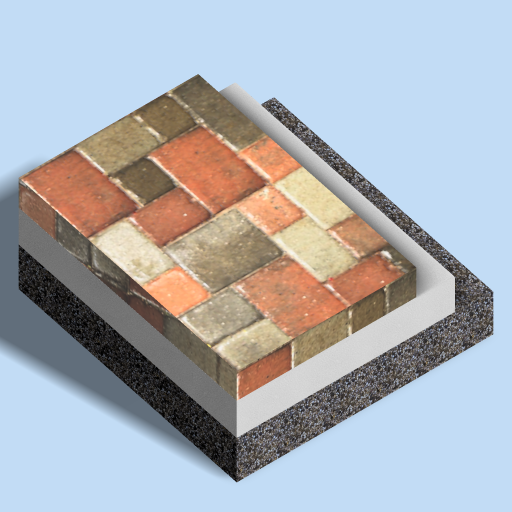
# Autodesk Inventor part: 부품1
Saved by Autodesk Inventor 2024.1 (Build 281209000, 209)
## iProperties
Created: 2024-01-18
Part Number: 부품1
Material: 일반
Document SubType Name: Modeling
Designer: likek
Density: 1 g/cm^3
Appearance: 기본값
Author: likek
Autodesk Inventor part; units mm, degrees
ref_plane "YZ Plane" through (0, 0, 0) normal (1, 0, 0) x (0, 1, 0)
ref_plane "XZ Plane" through (0, 0, 0) normal (0, 1, 0) x (-1, 0, 0)
ref_plane "XY Plane" through (0, 0, 0) normal (0, 0, 1) x (1, 0, 0)
sketch "스케치1" plane through (0, 0, 0) normal (0, 0, 1) x (1, 0, 0)
  line L0 (0, 0) -> (0, 150)
  line L1 (0, 150) -> (-850, 377.7568)
  line L2 (-850, 377.7568) -> (-850, 227.7568)
  line L3 (-850, 227.7568) -> (0, 0)
  line L4 (-311.1275, 0) -> (112.1526, 0)
  line L5 (-850, 377.7568) -> (-850, 602.7568)
  line L6 (-850, 602.7568) -> (0, 375)
  line L7 (0, 375) -> (0, 150)
  line L8 (-850, 502.7568) -> (0, 275)
  line L9 (-850, 602.7568) -> (-850, 612.7568)
  line L10 (-850, 612.7568) -> (0, 385)
  line L11 (0, 385) -> (0, 375)
  point P0 (0, 75)
  dimension "d0" = 150
  dimension "d1" = 150
  dimension "d2" = 15
  dimension "d3" = 850
  dimension "d4" = 125
  dimension "d5" = 100
  dimension "d12" = 10
  dimension "d13" = 10
  constraints: 24 end point, 5 parallel, 3 vertical, 2 point on line, 1 horizontal, 1 midpoint
  measures "d0" distance of L0.start L0.end
  measures "d1" distance of L1.end L2.end
  measures "d2" angle of L3 L4
  measures "d3" distance from line of point (0, 75) L2
  measures "d4" distance of L1.end L8.start
  measures "d5" distance of L5.end L8.start
  measures "d12" distance of L5.end L9.end
  measures "d13" distance of L10.end L6.end
extrude "돌출1" add sketch "스케치1" against normal blind 1000 contours L3 L2 L1 L0
extrude "돌출2" add sketch "스케치1" against normal blind 850 separate body contours L1 L5 L8 L7
extrude "돌출3" add sketch "스케치1" against normal blind 700 separate body contours L8 L5 L6 L7
fillet "모깎기2" radius 10 2 edges at (-425, 263.8784, -1000) (-425, 388.8784, -850)
